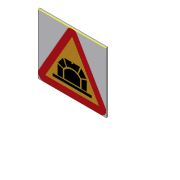
# Autodesk Inventor part: tunnel
Saved by Autodesk Inventor 2018 (Build 220112000, 112)
## iProperties
Created: 2017-08-24
Part Number: tunnel
Material: Generic
Document SubType Name: Modeling
Designer: Platform
Density: 1 g/cm^3
Appearance: Default
Author: Platform
Autodesk Inventor part; units mm, degrees
ref_plane "YZ Plane" through (0, 0, 0) normal (1, 0, 0) x (0, 1, 0)
ref_plane "XZ Plane" through (0, 0, 0) normal (0, 1, 0) x (-1, 0, 0)
ref_plane "XY Plane" through (0, 0, 0) normal (0, 0, 1) x (1, 0, 0)
sketch "Sketch4" plane through (0, 0, 0) normal (0, 0, 1) x (1, 0, 0)
  line L0 (-40, 35.4999) -> (40, 35.4999)
  line L1 (40, 35.4999) -> (40, -35.5001)
  line L2 (40, -35.5001) -> (-40, -35.5001)
  line L3 (-40, -35.5001) -> (-40, 35.4999)
  point P0 (0, 0)
  dimension "d40" = 80
  dimension "d43" = 71
  constraints: 8 end point, 2 parallel, 1 horizontal, 1 perpendicular
  measures "d40" distance between parallel lines of L1 L3
  measures "d43" distance between parallel lines of L0 L2
extrude "Extrusion2" add sketch "Sketch4" against normal blind 2
sketch "Sketch5" plane through (0, 0, 0) normal (0, 0, 1) x (1, 0, 0)
  line L0 (-40, 35.4999) -> (40, 35.4999) projected
  line L1 (-40, 35.4999) -> (39.8942, 35.4999) construction
  line L2 (39.8942, 35.4999) -> (39.8942, -35.3996) construction
  line L3 (39.8942, -35.3996) -> (-40, -35.3996) construction
  line L4 (-40, -35.3996) -> (-40, 35.4999) construction
  point P0 (0, 0)
  constraints: 2 other
body "Solid2"
